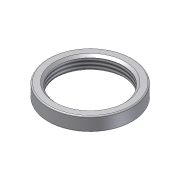
# Autodesk Inventor part: 13536_Ring
Saved by Autodesk Inventor 2013 (Build 170138000, 138)
## iProperties
Category: Pneumatics
Shininess: 64.0
Length Units: 11269
Angle Units: 11279
Time Units: 11290
Mass Units: 11283
Length Display Precision: 3
Angle Display Precision: 2
Compacted: True
Part Number: 13536_Ring
Document SubType Name: Modeling
Created: 2005-01-09
Manufacturer: Standard
Standards Organization: Custom
Density: 1 g/cm^3
Project: FIRST
Description: Retaining Ring for Secondary Regulator
Vendor: Monnier
Material: Generic
Density: 0.0
Volumn: 0.0
Area: 0.0
PropertySet Name: Model Information
Control State: 0
Master: False
Checked Out: False
Title: Retaining Ring - Secondary Regulator
Author: Autodesk, Inc.
Autodesk Inventor part; units mm, degrees
ref_plane "YZ Plane" through (0, 0, 0) normal (1, 0, 0) x (0, 1, 0)
ref_plane "XZ Plane" through (0, 0, 0) normal (0, 1, 0) x (-1, 0, 0)
ref_plane "XY Plane" through (0, 0, 0) normal (0, 0, 1) x (1, 0, 0)
sketch "Sketch1" plane through (0, 0, 0) normal (0, 0, 1) x (1, 0, 0)
  circle A0 centre (0, 0) radius 18.5
  circle A1 centre (0, 0) radius 14.5
  dimension "d0" = 37
  dimension "d1" = 29
  constraints: 2 centre point, 2 coincident
  measures "d0" diameter of A0
  measures "d1" diameter of A1
extrude "Extrusion1" add sketch "Sketch1" along normal blind 6.2
thread "Thread1" size "M30x1.5" class "6H" standard "ANSI Metric M Profile" full length
chamfer "Chamfer1" distance 1 angle 45 2 edges at (-14.5, 0, 6.2) (-14.5, 0, 0)
fillet "Fillet1" radius 0.5 2 edges at (-18.5, 0, 6.2) (-18.5, 0, 0)
body "Solid1"
